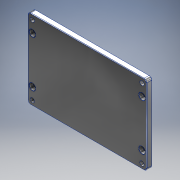
# Autodesk Inventor part: Conecting plate 1
Saved by Autodesk Inventor 2022 (Build 260153000, 153)
## iProperties
Created: 2022-11-11
Part Number: Conecting plate 1
Material: Aluminum 6061
Document SubType Name: Modeling
Designer: SimonD
Density: 2.7 g/cm^3
Appearance: Aluminum - Flat
Author: SimonD
Autodesk Inventor part; units mm, degrees
ref_plane "YZ Plane" through (0, 0, 0) normal (1, 0, 0) x (0, 1, 0)
ref_plane "XZ Plane" through (0, 0, 0) normal (0, 1, 0) x (-1, 0, 0)
ref_plane "XY Plane" through (0, 0, 0) normal (0, 0, 1) x (1, 0, 0)
sketch "Sketch1" plane through (0, 0, 0) normal (0, 0, 1) x (1, 0, 0)
  line L0 (-63.875, 42.75) -> (63.875, 42.75)
  line L1 (63.875, 42.75) -> (63.875, -42.75)
  line L2 (63.875, -42.75) -> (-63.875, -42.75)
  line L3 (-63.875, -42.75) -> (-63.875, 42.75)
  line L4 (-63.875, 42.75) -> (63.875, -42.75) construction
  line L5 (63.875, 42.75) -> (-63.875, -42.75) construction
  point P0 (0, 0)
  dimension "d0" = 85.5
  dimension "d1" = 127.75
  constraints: 12 end point, 2 midpoint, 2 parallel, 1 horizontal, 1 perpendicular
  measures "d0" distance between parallel lines of L2 L0
  measures "d1" distance between parallel lines of L1 L3
extrude "Extrusion1" add sketch "Sketch1" along normal blind 6
sketch "Sketch2" plane through (0, 0, 6) normal (0, 0, 1) x (1, 0, 0)
  point P0 (0, 0)
  point P1 (-59, 25)
  point P2 (-59, -25)
  point P3 (59, -25)
  point P4 (59, 25)
  dimension "d4" = 59
  dimension "d5" = 25
  dimension "d6" = 25
  dimension "d7" = 59
  measures "d4" horizontal distance of point (-59, 25) point (0, 0)
  measures "d5" vertical distance of point (-59, 25) point (0, 0)
  measures "d6" vertical distance of point (-59, -25) point (0, 0)
  measures "d7" horizontal distance of point (59, -25) point (0, 0)
fillet "Fillet1" radius 3 4 edges at (-63.875, 42.75, 3) (-63.875, -42.75, 3) (63.875, -42.75, 3) (63.875, 42.75, 3)
hole "Hole1" at (-59, 25, 6) at (-59, -25, 6) at (59, -25, 6) at (59, 25, 6) direction (0, 0, -1) diameter 4 end through all counterbore diameter 7 counterbore depth 4.1
chamfer "Chamfer1" distance 0.5 angle 45 16 edges at (0, 42.75, 0) (-62.9963, 41.8713, 0) (-63.875, 0, 0) (-62.9963, -41.8713, 0) (0, -42.75, 0) (62.9963, -41.8713, 0) (63.875, 0, 0) (62.9963, 41.8713, 0) (0, 42.75, 6) (-62.9963, 41.8713, 6) (-63.875, 0, 6) (-62.9963, -41.8713, 6) (0, -42.75, 6) (62.9963, -41.8713, 6) (63.875, 0, 6) (62.9963, 41.8713, 6)
chamfer "Chamfer2" distance 0.2 angle 45 8 edges at (-59, -21.5, 6) (59, -21.5, 6) (-59, 28.5, 6) (59, 28.5, 6) (-59, -23, 0) (59, -23, 0) (-59, 27, 0) (59, 27, 0)
sketch "Sketch3" plane through (0, 0, 6) normal (0, 0, 1) x (1, 0, 0)
  arc A0 (-60.875, 42.75) -> (-63.875, 39.75) centre (-60.875, 39.75) ccw projected
  arc A1 (63.875, 39.75) -> (60.875, 42.75) centre (60.875, 39.75) ccw projected
  arc A2 (60.875, -42.75) -> (63.875, -39.75) centre (60.875, -39.75) ccw projected
  arc A3 (-63.875, -39.75) -> (-60.875, -42.75) centre (-60.875, -39.75) ccw projected
  point P0 (0, 0)
  point P1 (-59, -37.5)
  point P2 (-59, 37.5)
  point P3 (59, 37.5)
  point P4 (59, -37.5)
  dimension "d29" = 37.5
  dimension "d30" = 37.5
  measures "d29" vertical distance of point (-59, -37.5) point (0, 0)
  measures "d30" vertical distance of point (-59, 37.5) point (0, 0)
hole "Hole2" at (-59, 37.5, 6) at (59, -37.5, 6) at (59, 37.5, 6) at (-59, -37.5, 6) direction (0, 0, -1) diameter 4.6 end through all
body "Solid1"
